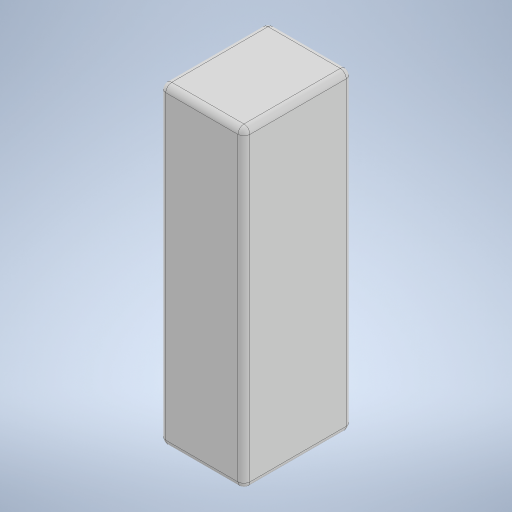
# Autodesk Inventor part: li-pol_520
Saved by Autodesk Inventor 2023 (Build 270158000, 158)
## iProperties
Created: 2024-05-17
Part Number: li-pol_520
Material: Ogólny
Document SubType Name: Modeling
Designer: kamil
Density: 1 g/cm^3
Appearance: Domyślna
Author: kamil
Autodesk Inventor part; units mm, degrees
ref_plane "YZ Plane" through (0, 0, 0) normal (1, 0, 0) x (0, 1, 0)
ref_plane "XZ Plane" through (0, 0, 0) normal (0, 1, 0) x (-1, 0, 0)
ref_plane "XY Plane" through (0, 0, 0) normal (0, 0, 1) x (1, 0, 0)
sketch "Szkic1" plane through (0, 0, 0) normal (0, 1, 0) x (-1, 0, 0)
  line L0 (2.2782, 2.7647) -> (-11.7218, 2.7647)
  line L1 (-11.7218, 2.7647) -> (-11.7218, -15.2353)
  line L2 (-11.7218, -15.2353) -> (2.2782, -15.2353)
  line L3 (2.2782, -15.2353) -> (2.2782, 2.7647)
  point P0 (0, 0)
  dimension "d0" = 14
  dimension "d1" = 18
  constraints: 8 end point, 2 parallel, 1 horizontal, 1 perpendicular
  measures "d0" distance of L2.end L1.end
  measures "d1" distance of L1.end L0.end
extrude "Wyciągnięcie proste1" add sketch "Szkic1" along normal blind 52
fillet "Zaokrąglenie1" radius 1 4 edges at (-2.2782, 26, -15.2353) (11.7218, 26, -15.2353) (-2.2782, 26, 2.7647) (11.7218, 26, 2.7647)
fillet "Zaokrąglenie2" radius 1 16 edges at (-1.9853, 0, 2.4719) (4.7218, 0, 2.7647) (11.429, 0, 2.4719) (11.7218, 0, -6.2353) (11.429, 0, -14.9424) (4.7218, 0, -15.2353) (-1.9853, 0, -14.9424) (-2.2782, 0, -6.2353) (-1.9853, 52, 2.4719) (4.7218, 52, 2.7647) (11.429, 52, 2.4719) (11.7218, 52, -6.2353) (11.429, 52, -14.9424) (4.7218, 52, -15.2353) (-1.9853, 52, -14.9424) (-2.2782, 52, -6.2353)
